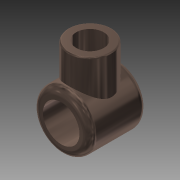
# Autodesk Inventor part: suporte-barra
Saved by Autodesk Inventor 2015 (Build 190159000, 159)
## iProperties
Created: 2016-08-11
Part Number: suporte-barra
Material: Ogólny
Document SubType Name: Modeling
Designer: EriveltonDell
Density: 1 g/cm^3
Appearance: Gunmetal - Antique Polished
Author: EriveltonDell
Autodesk Inventor part; units mm, degrees
ref_plane "YZ Plane" through (0, 0, 0) normal (1, 0, 0) x (0, 1, 0)
ref_plane "XZ Plane" through (0, 0, 0) normal (0, 1, 0) x (-1, 0, 0)
ref_plane "XY Plane" through (0, 0, 0) normal (0, 0, 1) x (1, 0, 0)
sketch "Sketch1" plane through (0, 0, 0) normal (0, 1, 0) x (-1, 0, 0)
  circle A0 centre (0, 0) radius 12.7
  circle A1 centre (0, 0) radius 20
  dimension "d0" = 25.4
  dimension "d1" = 40
  constraints: 2 centre point, 2 coincident
  measures "d0" diameter of A0
  measures "d1" diameter of A1
extrude "Extrusion1" add sketch "Sketch1" along normal mid plane 40
fillet "Fillet2" radius 5 2 edges at (20, 20, 0) (20, -20, 0)
sketch "Sketch6" plane through (0, 0, 0) normal (0, 0, 1) x (1, 0, 0)
  circle A0 centre (0, 0) radius 15
  dimension "d33" = 30
  constraints: 1 centre point, 1 coincident
  measures "d33" diameter of A0
extrude "Extrusion6" add sketch "Sketch6" along normal blind 40
sketch "Sketch7" plane through (0, 0, 0) normal (0, 1, 0) x (-1, 0, 0)
  circle A0 centre (0, 0) radius 12.7
  constraints: 1 centre point, 1 coincident
extrude "Extrusion7" cut sketch "Sketch7" along normal through all both and the other way through all
hole "Hole2" at (0, 0, 40) direction (0, 0, -1) diameter 19 depth 15
fillet "Fillet3" radius 1 1 edges at (-15, 0, 40)
body "Solid1"
